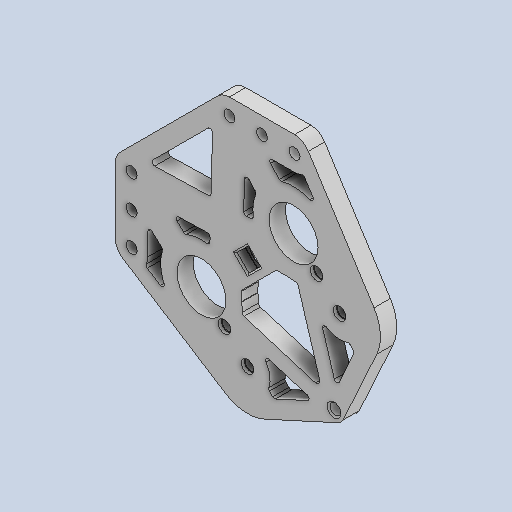
# Autodesk Inventor part: motorplate
Saved by Autodesk Inventor 2022 (Build 260153000, 153)
## iProperties
Created: 2022-03-17
Part Number: motorplate
Material: Generic
Document SubType Name: Modeling
Designer: zac-h
Density: 1 g/cm^3
Appearance: Default
Author: zac-h
## iProperties of the stored document motorplate_3DPrint.ipt
Created: 2022-03-19
Part Number: motorplate_3DPrint
Material: Generic
Document SubType Name: Modeling
Designer: zac-h
Density: 1 g/cm^3
Appearance: Default
Author: zac-h
Autodesk Inventor part; units mm, degrees
ref_plane "YZ Plane" through (0, 0, 0) normal (1, 0, 0) x (0, 1, 0)
ref_plane "XZ Plane" through (0, 0, 0) normal (0, 1, 0) x (-1, 0, 0)
ref_plane "XY Plane" through (0, 0, 0) normal (0, 0, 1) x (1, 0, 0)
sketch "Sketch1" plane through (0, 0, 0) normal (0, 0, 1) x (1, 0, 0)
  line L0 (-54.9162, 38.4967) -> (-54.9162, 12.4519) projected
  arc A0 (-54.9162, -18.4488) -> (-54.6412, -19.1376) centre (-53.9162, -18.4488) ccw projected
  line L1 (-54.6412, -19.1376) -> (-23.6992, -51.7087) projected
  arc A1 (-23.6992, -51.7087) -> (-14.0094, -54.6745) centre (-16.228, -44.6112) ccw projected
  line L2 (-14.0094, -54.6745) -> (-0.0667, -51.6007) projected
  arc A2 (-0.0667, -51.6007) -> (0.1266, -51.5369) centre (-0.282, -50.6241) ccw projected
  line L3 (0.1266, -51.5369) -> (17.6889, -43.6752) projected
  line L4 (43.6752, -17.6889) -> (51.5369, -0.1266) projected
  arc A3 (51.5369, -0.1266) -> (51.6007, 0.0667) centre (50.6241, 0.282) ccw projected
  line L5 (51.6007, 0.0667) -> (54.6745, 14.0094) projected
  arc A4 (54.6745, 14.0094) -> (51.7087, 23.6992) centre (44.6112, 16.228) ccw projected
  line L6 (51.7087, 23.6992) -> (19.1376, 54.6412) projected
  arc A5 (19.1376, 54.6412) -> (18.4488, 54.9162) centre (18.4488, 53.9162) ccw projected
  line L7 (0.0011, 54.9162) -> (-8.4105, 54.9162) projected
  circle A6 centre (14.5893, 21.3317) radius 9.525
  line L8 (-3.3712, 3.3712) -> (68.4985, -68.4985) construction
  circle A7 centre (30.3259, -30.3259) radius 3.8901
  line L9 (30.3259, -30.3259) -> (-3.3712, 3.3712) construction
  line L10 (14.5893, 21.3317) -> (32.5498, 3.3712) construction
  circle A8 centre (14.5893, 21.3317) radius 2.132
  circle A9 centre (23.5696, 12.3514) radius 2.132
  circle A10 centre (32.5498, 3.3712) radius 2.132
  line L11 (14.9688, 48.5312) -> (-10.4312, 48.5312) construction
  line L12 (14.9688, 42.1462) -> (-10.4312, 42.1462)
  line L13 (-10.4312, 54.9162) -> (14.9688, 54.9162)
  arc A11 (14.9688, 42.1462) -> (14.9688, 54.9162) centre (14.9688, 48.5312) ccw
  arc A12 (-10.4312, 54.9162) -> (-10.4312, 42.1462) centre (-10.4312, 48.5312) ccw
  line L14 (43.7752, 14.5965) -> (33.2607, 25.111)
  arc A13 (33.2607, 25.111) -> (-1.2806, 31.8696) centre (14.5893, 21.3317) ccw
  arc A14 (-1.2806, 31.8696) -> (-31.8696, 1.2806) centre (-3.3712, 3.3712) ccw
  arc A15 (-31.8696, 1.2806) -> (-25.111, -33.2607) centre (-21.3317, -14.5893) ccw
  line L15 (-25.111, -33.2607) -> (-14.5965, -43.7752)
  arc A16 (-14.5965, -43.7752) -> (8.8742, -22.4471) centre (-3.3712, -32.5498) ccw
  arc A17 (8.8742, -22.4471) -> (22.4471, -8.8742) centre (-3.3712, 3.3712) ccw
  arc A18 (22.4471, -8.8742) -> (43.7752, 14.5965) centre (32.5498, 3.3712) ccw
  line L16 (46.9883, -3.2279) -> (33.864, -31.943)
  line L17 (45.9291, 11.9158) -> (20.35, 51.9679)
  line L18 (-11.9158, -45.9291) -> (-51.9679, -20.35)
  circle A19 centre (-12.3514, -23.5696) radius 2.132
  circle A20 centre (-3.3712, -32.5498) radius 2.132
  arc A21 (-54.9162, -14.9688) -> (-42.1462, -14.9688) centre (-48.5312, -14.9688) ccw
  arc A22 (-42.1462, 10.4312) -> (-54.9162, 10.4312) centre (-48.5312, 10.4312) ccw
  line L19 (3.2279, -46.9883) -> (31.943, -33.864)
  line L20 (-53.0461, 14.9461) -> (-14.9461, 53.0461)
  circle A23 centre (-21.3317, -14.5893) radius 9.525
  arc A24 (17.6889, -43.6752) -> (30.0935, -35.8334) centre (-3.3712, 3.3712) ccw projected
  arc A25 (30.0935, -35.8334) -> (29.6251, -33.7616) centre (29.3145, -34.9207) ccw projected
  line L21 (29.6251, -33.7616) -> (27.4682, -33.1836) projected
  line L22 (27.4682, -33.1836) -> (26.4222, -29.2799) projected
  line L23 (26.4222, -29.2799) -> (29.2799, -26.4222) projected
  line L24 (29.2799, -26.4222) -> (33.1836, -27.4682) projected
  line L25 (33.1836, -27.4682) -> (33.7616, -29.6251) projected
  arc A26 (33.7616, -29.6251) -> (35.8334, -30.0935) centre (34.9207, -29.3145) ccw projected
  arc A27 (35.8334, -30.0935) -> (43.6752, -17.6889) centre (-3.3712, 3.3712) ccw projected
  arc A28 (7.8958, -33.0248) -> (33.0248, -7.8958) centre (-3.3712, 3.3712) ccw projected
  arc A29 (-10.1064, -39.285) -> (5.7833, -35.1808) centre (-3.3712, -32.5498) ccw projected
  line L26 (-10.1064, -39.285) -> (-16.8416, -32.5498) projected
  arc A30 (31.8591, 17.8778) -> (-17.8778, -31.8591) centre (-3.3712, 3.3712) ccw projected
  line L27 (32.5498, 16.8416) -> (39.285, 10.1064) projected
  arc A31 (35.1808, -5.7833) -> (39.285, 10.1064) centre (32.5498, 3.3712) ccw projected
  arc A32 (-38.4967, 54.9162) -> (-54.9162, 38.4967) centre (-38.4967, 38.4967) ccw projected
  arc A33 (-16.8416, -32.5498) -> (-17.8778, -31.8591) centre (-19.0866, -34.7949) ccw projected
  arc A34 (31.8591, 17.8778) -> (32.5498, 16.8416) centre (34.7949, 19.0866) ccw projected
  arc A35 (35.1808, -5.7833) -> (33.0248, -7.8958) centre (36.0578, -8.8347) ccw projected
  arc A36 (7.8958, -33.0248) -> (5.7833, -35.1808) centre (8.8347, -36.0578) ccw projected
  circle A37 centre (30.3259, -30.3259) radius 2.132
  line L28 (-8.4105, 54.9162) -> (-8.4105, 53.2312) projected
  line L29 (-8.4105, 53.2312) -> (-7.7176, 53.2312) projected
  line L30 (-7.7176, 53.2312) -> (-5.0041, 48.5312) projected
  line L31 (-5.0041, 48.5312) -> (-7.7176, 43.8312) projected
  line L32 (-7.7176, 43.8312) -> (-13.1447, 43.8312) projected
  line L33 (-13.1447, 43.8312) -> (-15.8583, 48.5312) projected
  line L34 (-15.8583, 48.5312) -> (-13.1447, 53.2312) projected
  line L35 (-13.1447, 53.2312) -> (-12.4519, 53.2312) projected
  line L36 (-12.4519, 53.2312) -> (-12.4519, 54.9162) projected
  line L37 (-12.4519, 54.9162) -> (-38.4967, 54.9162) projected
  line L38 (-54.9162, 12.4519) -> (-53.2312, 12.4519) projected
  line L39 (-53.2312, 12.4519) -> (-53.2312, 13.1447) projected
  line L40 (-53.2312, 13.1447) -> (-48.5312, 15.8583) projected
  line L41 (-48.5312, 15.8583) -> (-43.8312, 13.1447) projected
  line L42 (-43.8312, 13.1447) -> (-43.8312, 7.7176) projected
  line L43 (-43.8312, 7.7176) -> (-48.5312, 5.0041) projected
  line L44 (-48.5312, 5.0041) -> (-53.2312, 7.7176) projected
  line L45 (-53.2312, 7.7176) -> (-53.2312, 8.4105) projected
  line L46 (-53.2312, 8.4105) -> (-54.9162, 8.4105) projected
  line L47 (-54.9162, 8.4105) -> (-54.9162, -0.2481) projected
  line L48 (-54.9162, -0.2481) -> (-53.2312, -0.2481) projected
  line L49 (-53.2312, -0.2481) -> (-53.2312, 0.4447) projected
  line L50 (-53.2312, 0.4447) -> (-48.5312, 3.1583) projected
  line L51 (-48.5312, 3.1583) -> (-43.8312, 0.4447) projected
  line L52 (-43.8312, 0.4447) -> (-43.8312, -4.9824) projected
  line L53 (-43.8312, -4.9824) -> (-48.5312, -7.6959) projected
  line L54 (-48.5312, -7.6959) -> (-53.2312, -4.9824) projected
  line L55 (-53.2312, -4.9824) -> (-53.2312, -4.2895) projected
  line L56 (-53.2312, -4.2895) -> (-54.9162, -4.2895) projected
  line L57 (-54.9162, -4.2895) -> (-54.9162, -12.9481) projected
  line L58 (-54.9162, -12.9481) -> (-53.2312, -12.9481) projected
  line L59 (-53.2312, -12.9481) -> (-53.2312, -12.2553) projected
  line L60 (-53.2312, -12.2553) -> (-48.5312, -9.5417) projected
  line L61 (-48.5312, -9.5417) -> (-43.8312, -12.2553) projected
  line L62 (-43.8312, -12.2553) -> (-43.8312, -17.6824) projected
  line L63 (-43.8312, -17.6824) -> (-48.5312, -20.3959) projected
  line L64 (-48.5312, -20.3959) -> (-53.2312, -17.6824) projected
  line L65 (-53.2312, -17.6824) -> (-53.2312, -16.9895) projected
  line L66 (-53.2312, -16.9895) -> (-54.9162, -16.9895) projected
  line L67 (-54.9162, -16.9895) -> (-54.9162, -18.4488) projected
  line L68 (18.4488, 54.9162) -> (16.9895, 54.9162) projected
  line L69 (16.9895, 54.9162) -> (16.9895, 53.2312) projected
  line L70 (16.9895, 53.2312) -> (17.6824, 53.2312) projected
  line L71 (17.6824, 53.2312) -> (20.3959, 48.5312) projected
  line L72 (20.3959, 48.5312) -> (17.6824, 43.8312) projected
  line L73 (17.6824, 43.8312) -> (12.2553, 43.8312) projected
  line L74 (12.2553, 43.8312) -> (9.5417, 48.5312) projected
  line L75 (9.5417, 48.5312) -> (12.2553, 53.2312) projected
  line L76 (12.2553, 53.2312) -> (12.9481, 53.2312) projected
  line L77 (12.9481, 53.2312) -> (12.9481, 54.9162) projected
  line L78 (12.9481, 54.9162) -> (4.2895, 54.9162) projected
  line L79 (4.2895, 54.9162) -> (4.2895, 53.2312) projected
  line L80 (4.2895, 53.2312) -> (4.9824, 53.2312) projected
  line L81 (4.9824, 53.2312) -> (7.6959, 48.5312) projected
  line L82 (7.6959, 48.5312) -> (4.9824, 43.8312) projected
  line L83 (4.9824, 43.8312) -> (-0.4447, 43.8312) projected
  line L84 (-0.4447, 43.8312) -> (-3.1583, 48.5312) projected
  line L85 (-3.1583, 48.5312) -> (-0.4447, 53.2312) projected
  line L86 (-0.4447, 53.2312) -> (0.0011, 53.2312) projected
  line L87 (0.0011, 53.2312) -> (0.0011, 54.9162) projected
  circle A38 centre (14.9688, 48.5312) radius 2.132
  circle A39 centre (2.2688, 48.5312) radius 2.132
  circle A40 centre (-10.4312, 48.5312) radius 2.132
  circle A41 centre (-48.5312, 10.4312) radius 2.132
  circle A42 centre (-48.5312, -14.9688) radius 2.1673
  circle A43 centre (-48.5312, -2.2688) radius 2.1673
  line L88 (-54.9162, -16.9895) -> (-54.9162, -12.9481)
  line L89 (-54.9162, -4.2895) -> (-54.9162, 10.4312)
  line L90 (16.9895, 54.9162) -> (-12.4519, 54.9162)
  line L91 (-54.9162, 12.5632) -> (-54.9162, 10.4312)
  point P0 (0, 0)
  point P1 (-54.9162, 10.4312)
  point P2 (-3.3712, 3.3712)
  point P3 (-3.3712, 3.3712)
  point P4 (16.9895, 54.588)
  point P5 (-12.4519, 54.588)
  point P6 (30.454, -34.5445)
  point P7 (34.5445, -30.454)
  point P8 (-54.588, -16.9895)
  point P9 (-54.588, 12.4519)
  dimension "d9" = 19.05
  dimension "d16" = 4.264
  dimension "d19" = 12.7
  dimension "d57" = 4.264
  dimension "d61" = 4.264
  dimension "d62" = 4.264
  constraints: 36 end point, 25 point on circle, 24 centre point, 13 symmetric about line, 12 tangent, 7 coincident, 3 collinear, 2 vertical, 1 horizontal, 1 midpoint, 1 parallel, 1 point on line, 14 other
  measures "d9" diameter of A6
  measures "d16" diameter of A8
  measures "d19" distance of A8.centre A9.centre
  measures "d57" diameter of A37
  measures "d61" diameter of A38
  measures "d62" diameter of A41
extrude "Extrusion1" add sketch "Sketch1" along normal blind 6.35 contours L38 L39 L40 L41 L42 L43 L44 L45 L46 L89 A22 | A22 L20 A12 L12 A11 L17 A18 L14 A13 A30 A15 L15 A16 L18 A21 L66 L65 L64 L63 L62 L61 L60 L59 L58 L57 L56 L55 L54 L53 L52 L51 L50 L49 L48 L47 L46 L45 L44 L43 L42 L41 L40 L39 L38 | L36 L35 L34 L33 L32 L31 L30 L29 L28 L7 L87 L86 L85 L84 L83 L82 L81 L80 L79 L13 L77 L76 L75 L74 L73 L72 L71 L70 L69 A11 L12 A12 | A12 L13 L28 L29 L30 L31 L32 L33 L34 L35 L36 | L48 L49 L50 L51 L52 L53 L54 L55 L56 L89 | L13 L79 L80 L81 L82 L83 L84 L85 L86 L87 | L58 L59 L60 L61 L62 L63 L64 L65 L66 A21 L88 | L13 A11 L69 L70 L71 L72 L73 L74 L75 L76 L77 | A18 A28 A35 A31 L27 A34 A30 A13 L14 | L16 A26 A7 L25 L24 L23 L22 L21 A25 L19 A16 A28 A18 | A28 A16 A17 A18 | A18 A17 A16 A28 A36 A29 L26 A33 A30 A15 A14 A13 A34 L27 A31 A35 | L16 A7 A26 | A16 L15 A15 A30 A33 L26 A29 A36 A28 | A7 A25 L21 L22 L23 L24 L25 A26 | A26 L25 A7 | A13 A14 A15 A30 | L19 A25 A7 | A7 L24 L25 | A7 L21 A25 | L24 A7 | L21 L22 A7 | A7 L23 L24 | A7 L22 | L23 A7 | L22 L23 A7
sketch "Sketch2" plane through (0, 0, 6.35) normal (0, 0, 1) x (1, 0, 0)
  circle A0 centre (-48.5312, -14.9688) radius 2.132 projected
  arc A1 (20.35, 51.9679) -> (14.9688, 54.9162) centre (14.9688, 48.5312) ccw projected
  arc A2 (-54.9162, -14.9688) -> (-51.9679, -20.35) centre (-48.5312, -14.9688) ccw projected
  line L0 (-51.9679, -20.35) -> (-11.9158, -45.9291) projected
  arc A3 (-11.9158, -45.9291) -> (3.2279, -46.9883) centre (-3.3712, -32.5498) ccw projected
  line L1 (3.2279, -46.9883) -> (31.943, -33.864) projected
  arc A4 (31.943, -33.864) -> (33.864, -31.943) centre (30.3259, -30.3259) ccw projected
  line L2 (33.864, -31.943) -> (46.9883, -3.2279) projected
  arc A5 (46.9883, -3.2279) -> (45.9291, 11.9158) centre (32.5498, 3.3712) ccw projected
  line L3 (45.9291, 11.9158) -> (20.35, 51.9679) projected
  circle A6 centre (-21.3317, -14.5893) radius 9.525 projected
  circle A7 centre (-3.3712, -32.5498) radius 2.132 projected
  circle A8 centre (-12.3514, -23.5696) radius 2.132 projected
  circle A9 centre (32.5498, 3.3712) radius 2.132 projected
  circle A10 centre (23.5696, 12.3514) radius 2.132 projected
  circle A11 centre (14.5893, 21.3317) radius 9.525 projected
  circle A12 centre (32.5498, 3.3712) radius 2.4614
  circle A13 centre (23.5696, 12.3514) radius 2.4614
  circle A14 centre (-3.3712, -32.5498) radius 2.132 projected
  circle A15 centre (-3.3712, -32.5498) radius 2.4614
  circle A16 centre (-12.3514, -23.5696) radius 2.4614
  line L4 (14.9688, 54.9162) -> (-10.4312, 54.9162) projected
  arc A17 (-10.4312, 54.9162) -> (-14.9461, 53.0461) centre (-10.4312, 48.5312) ccw projected
  line L5 (-14.9461, 53.0461) -> (-53.0461, 14.9461) projected
  arc A18 (-53.0461, 14.9461) -> (-54.9162, 10.4312) centre (-48.5312, 10.4312) ccw projected
  line L6 (-54.9162, 10.4312) -> (-54.9162, -14.9688) projected
  dimension "d26" = 4.9228
  constraints: 4 centre point, 4 coincident, 3 equal radius
  measures "d26" diameter of A12
extrude "Extrusion2" cut sketch "Sketch2" against normal blind 1.27 contours A7 | A8 | A9 | A10 | A12 | A13 | A15 | A16
sketch "Sketch3" plane through (0, 0, 6.35) normal (0, 0, 1) x (1, 0, 0)
  circle A0 centre (32.5498, 3.3712) radius 2.4614 projected
  circle A1 centre (-12.3514, -23.5696) radius 2.4614 projected
  circle A2 centre (23.5696, 12.3514) radius 2.4614 projected
  circle A3 centre (-3.3712, -32.5498) radius 2.4614 projected
  arc A4 (20.35, 51.9679) -> (14.9688, 54.9162) centre (14.9688, 48.5312) ccw projected
  arc A5 (-54.9162, -14.9688) -> (-51.9679, -20.35) centre (-48.5312, -14.9688) ccw projected
  line L0 (-51.9679, -20.35) -> (-11.9158, -45.9291) projected
  arc A6 (-11.9158, -45.9291) -> (3.2279, -46.9883) centre (-3.3712, -32.5498) ccw projected
  line L1 (3.2279, -46.9883) -> (31.943, -33.864) projected
  arc A7 (31.943, -33.864) -> (33.864, -31.943) centre (30.3259, -30.3259) ccw projected
  line L2 (33.864, -31.943) -> (46.9883, -3.2279) projected
  arc A8 (46.9883, -3.2279) -> (45.9291, 11.9158) centre (32.5498, 3.3712) ccw projected
  line L3 (45.9291, 11.9158) -> (20.35, 51.9679) projected
  circle A9 centre (-21.3317, -14.5893) radius 9.525 projected
  circle A10 centre (14.5893, 21.3317) radius 9.525 projected
  line L4 (-48.5559, 10.4559) -> (-10.4559, 48.5559)
  arc A11 (-10.4312, 48.5662) -> (-10.4559, 48.5559) centre (-10.4312, 48.5312) ccw
  line L5 (-10.4312, 48.5662) -> (14.9688, 48.5662)
  arc A12 (14.9983, 48.55) -> (14.9688, 48.5662) centre (14.9688, 48.5312) ccw
  line L6 (14.9983, 48.55) -> (40.5774, 8.498)
  arc A13 (41.2129, -0.5883) -> (40.5774, 8.498) centre (32.5498, 3.3712) ccw
  line L7 (41.2129, -0.5883) -> (28.4697, -28.4697)
  line L8 (28.4697, -28.4697) -> (0.5883, -41.2129)
  arc A14 (-8.498, -40.5774) -> (0.5883, -41.2129) centre (-3.3712, -32.5498) ccw
  line L9 (-8.498, -40.5774) -> (-48.55, -14.9983)
  arc A15 (-48.5662, -14.9688) -> (-48.55, -14.9983) centre (-48.5312, -14.9688) ccw
  line L10 (-48.5662, -14.9688) -> (-48.5662, 10.4312)
  arc A16 (-48.5559, 10.4559) -> (-48.5662, 10.4312) centre (-48.5312, 10.4312) ccw
  line L11 (-48.5662, 10.4312) -> (-48.5662, -14.9688) construction
  line L12 (-54.9162, 10.4312) -> (-54.9162, -14.9688)
  line L13 (-42.2162, -14.9688) -> (-42.2162, 10.4312)
  arc A17 (-42.2162, 10.4312) -> (-54.9162, 10.4312) centre (-48.5662, 10.4312) ccw
  arc A18 (-54.9162, -14.9688) -> (-42.2162, -14.9688) centre (-48.5662, -14.9688) ccw
  circle A19 centre (-21.3317, -14.5893) radius 15.875
  circle A20 centre (-12.3514, -23.5696) radius 8.8114
  circle A21 centre (-3.3712, -32.5498) radius 8.8114
  circle A22 centre (30.3259, -30.3259) radius 8.482
  circle A23 centre (32.5498, 3.3712) radius 8.8114
  circle A24 centre (23.5696, 12.3514) radius 8.8114
  circle A25 centre (14.5893, 21.3317) radius 15.875
  circle A26 centre (-10.4312, 48.5312) radius 2.132 projected
  circle A27 centre (14.9688, 48.5312) radius 2.132 projected
  line L14 (-10.4312, 48.5312) -> (14.9688, 48.5312) construction
  line L15 (-10.4312, 42.1812) -> (14.9688, 42.1812)
  line L16 (14.9688, 54.8812) -> (-10.4312, 54.8812)
  arc A28 (-10.4312, 54.8812) -> (-10.4312, 42.1812) centre (-10.4312, 48.5312) ccw
  arc A29 (14.9688, 42.1812) -> (14.9688, 54.8812) centre (14.9688, 48.5312) ccw
  line L17 (-21.3317, -14.5893) -> (14.5893, 21.3317) construction
  line L18 (-16.8416, -19.0795) -> (19.0795, 16.8416)
  line L19 (10.0992, 25.8218) -> (-25.8218, -10.0992)
  arc A30 (-25.8218, -10.0992) -> (-16.8416, -19.0795) centre (-21.3317, -14.5893) ccw
  arc A31 (19.0795, 16.8416) -> (10.0992, 25.8218) centre (14.5893, 21.3317) ccw
  line L20 (14.5893, 21.3317) -> (66.3854, -30.4643) construction
  line L21 (12.3443, 19.0866) -> (64.1403, -32.7094)
  line L22 (68.6304, -28.2193) -> (16.8344, 23.5768)
  arc A32 (16.8344, 23.5768) -> (12.3443, 19.0866) centre (14.5893, 21.3317) ccw
  arc A33 (64.1403, -32.7094) -> (68.6304, -28.2193) centre (66.3854, -30.4643) ccw
  line L23 (14.5893, 21.3317) -> (87.84, 21.3317) construction
  line L24 (-21.3317, -14.5893) -> (30.4643, -66.3854) construction
  line L25 (-23.5768, -16.8344) -> (28.2193, -68.6304)
  line L26 (32.7094, -64.1403) -> (-19.0866, -12.3443)
  arc A34 (-19.0866, -12.3443) -> (-23.5768, -16.8344) centre (-21.3317, -14.5893) ccw
  arc A35 (28.2193, -68.6304) -> (32.7094, -64.1403) centre (30.4643, -66.3854) ccw
  line L27 (-21.3317, -14.5893) -> (51.9189, -14.5893) construction
  line L28 (14.5893, 21.3317) -> (-10.4312, 48.5312) construction
  line L29 (19.2627, 25.6307) -> (-5.7578, 52.8302)
  line L30 (-15.1046, 44.2322) -> (9.9159, 17.0327)
  arc A36 (9.9159, 17.0327) -> (19.2627, 25.6307) centre (14.5893, 21.3317) ccw
  arc A37 (-5.7578, 52.8302) -> (-15.1046, 44.2322) centre (-10.4312, 48.5312) ccw
  line L31 (-21.3317, -14.5893) -> (-48.5662, 10.4312) construction
  line L32 (-17.0357, -9.9132) -> (-44.2701, 15.1074)
  line L33 (-52.8622, 5.755) -> (-25.6277, -19.2655)
  arc A38 (-25.6277, -19.2655) -> (-17.0357, -9.9132) centre (-21.3317, -14.5893) ccw
  arc A39 (-44.2701, 15.1074) -> (-52.8622, 5.755) centre (-48.5662, 10.4312) ccw
  circle A40 centre (30.3259, -30.3259) radius 2.132 projected
  line L34 (30.3259, -30.3259) -> (14.5893, 21.3317) construction
  line L35 (33.3631, -29.4007) -> (17.6265, 22.2569)
  line L36 (11.5521, 20.4065) -> (27.2887, -31.2511)
  arc A41 (27.2887, -31.2511) -> (33.3631, -29.4007) centre (30.3259, -30.3259) ccw
  arc A42 (17.6265, 22.2569) -> (11.5521, 20.4065) centre (14.5893, 21.3317) ccw
  line L37 (-21.3317, -14.5893) -> (30.3259, -30.3259) construction
  line L38 (-22.2569, -17.6265) -> (29.4007, -33.3631)
  line L39 (31.2511, -27.2887) -> (-20.4065, -11.5521)
  arc A43 (-20.4065, -11.5521) -> (-22.2569, -17.6265) centre (-21.3317, -14.5893) ccw
  arc A44 (29.4007, -33.3631) -> (31.2511, -27.2887) centre (30.3259, -30.3259) ccw
  circle A45 centre (-48.5312, 10.4312) radius 2.132 projected
  circle A46 centre (23.5696, 12.3514) radius 2.132 projected
  line L40 (-48.5312, 10.4312) -> (23.5696, 12.3514) construction
  line L41 (-48.3621, 4.0834) -> (23.7386, 6.0037)
  line L42 (23.4005, 18.6992) -> (-48.7002, 16.7789)
  arc A47 (-48.7002, 16.7789) -> (-48.3621, 4.0834) centre (-48.5312, 10.4312) ccw
  arc A48 (23.7386, 6.0037) -> (23.4005, 18.6992) centre (23.5696, 12.3514) ccw
  circle A49 centre (-12.3514, -23.5696) radius 2.132 projected
  line L43 (-10.4312, 48.5312) -> (-12.3514, -23.5696) construction
  line L44 (-16.7789, 48.7002) -> (-18.6992, -23.4005)
  line L45 (-6.0037, -23.7386) -> (-4.0834, 48.3621)
  arc A50 (-4.0834, 48.3621) -> (-16.7789, 48.7002) centre (-10.4312, 48.5312) ccw
  arc A51 (-18.6992, -23.4005) -> (-6.0037, -23.7386) centre (-12.3514, -23.5696) ccw
  line L46 (14.9688, 54.9162) -> (-10.4312, 54.9162) projected
  arc A52 (-10.4312, 54.9162) -> (-14.9461, 53.0461) centre (-10.4312, 48.5312) ccw projected
  line L47 (-14.9461, 53.0461) -> (-53.0461, 14.9461) projected
  arc A53 (-53.0461, 14.9461) -> (-54.9162, 10.4312) centre (-48.5312, 10.4312) ccw projected
  line L48 (-54.9162, 10.4312) -> (-54.9162, -14.9688) projected
  point P0 (0, 0)
  point P1 (-48.5662, -2.2688)
  point P2 (2.2688, 48.5312)
  point P3 (-3.3712, 3.3712)
  point P4 (40.4873, -4.5663)
  point P5 (4.5663, -40.4873)
  point P6 (2.0791, 34.9314)
  point P7 (-34.9489, -2.0791)
  point P8 (22.4576, -4.4971)
  point P9 (4.4971, -22.4576)
  point P10 (-12.4808, 11.3913)
  point P11 (-11.3913, 12.4808)
  point P12 (-18.0508, 0.9429)
  point P13 (-17.9456, 4.8935)
  point P14 (-32.7241, 4.4999)
  point P15 (-27.7501, -0.0697)
  point P16 (-36.3422, -9.4221)
  point P17 (-42.2162, -4.0256)
  point P18 (-43.2232, -18.4003)
  point P19 (-33.7957, -24.4211)
  point P20 (4.0382, 42.1812)
  point P21 (9.4124, 36.3389)
  point P22 (24.4211, 33.7957)
  point P23 (18.4161, 43.1984)
  point P24 (-4.5004, 32.7045)
  point P25 (-4.8935, 17.9456)
  point P26 (-0.9429, 18.0508)
  point P27 (0.0656, 27.7408)
  point P28 (-17.607, 17.607)
  point P29 (-16.9559, 42.056)
  point P30 (-42.056, 16.9559)
  point P31 (24.4007, 0.0198)
  point P32 (31.0711, -21.8767)
  point P33 (31.463, -21.9205)
  point P34 (38.329, -6.8981)
  point P35 (36.1168, -4.6859)
  point P36 (21.8767, -31.0711)
  point P37 (-0.0198, -24.4007)
  point P38 (4.6859, -36.1168)
  point P39 (6.8981, -38.329)
  point P40 (21.9205, -31.463)
  point P41 (-5.5797, -7.8176)
  point P42 (-5.6881, -11.8887)
  point P43 (-5.5273, -16.0848)
  point P44 (23.7272, -24.9967)
  point P45 (24.9967, -23.7272)
  point P46 (16.0848, 5.5273)
  point P47 (11.8887, 5.6881)
  point P48 (7.8176, 5.5797)
  dimension "d28" = 12.7
  dimension "d29" = 6.35
  dimension "d30" = 6.35
  dimension "d31" = 6.35
  dimension "d33" = 12.7
  dimension "d34" = 12.7
  dimension "d35" = 45
  dimension "d36" = 6.35
  dimension "d37" = 45
  dimension "d38" = 6.35
  dimension "d39" = 12.7
  dimension "d40" = 12.7
  dimension "d41" = 6.35
  dimension "d42" = 6.35
  dimension "d43" = 12.7
  dimension "d44" = 12.7
  constraints: 106 end point, 56 point on circle, 44 tangent, 35 centre point, 14 equal length, 11 midpoint, 6 equal radius, 3 horizontal, 7 other
  measures "d28" diameter of A18
  measures "d29" radial gap between concentric circles of A9 A19
  measures "d30" radial gap between concentric circles of A1 A20
  measures "d31" radial gap between concentric circles of A3 A21
  measures "d33" diameter of A29
  measures "d34" diameter of A31
  measures "d35" angle of L20 L23
  measures "d36" diameter of A33
  measures "d37" angle of L24 L27
  measures "d38" diameter of A35
  measures "d39" diameter of A37
  measures "d40" diameter of A39
  measures "d41" diameter of A42
  measures "d42" diameter of A44
  measures "d43" diameter of A48
  measures "d44" diameter of A51
extrude "Extrusion3" cut sketch "Sketch3" against normal through all contours L7 A22 L35 A23 L21 | A18 L13 L33 A19 L9 | L4 L44 L42 | L8 L26 A21 L38 A22 | A22 L39 A19 L45 L18 L41 A25 L36 | A25 L29 L15 A29 L6 | L41 L44 A19 L32 | L45 L30 A25 L42
fillet "Fillet1" radius 1 37 edges at (24.4007, 0.0198, 3.175) (31.0711, -21.8767, 3.175) (31.463, -21.9205, 3.175) (38.329, -6.8981, 3.175) (36.1168, -4.6859, 3.175) (-36.3422, -9.4221, 3.175) (-42.2162, -4.0256, 3.175) (-43.2232, -18.4003, 3.175) (-33.7957, -24.4211, 3.175) (4.0382, 42.1812, 3.175) (9.4124, 36.3389, 3.175) (24.4211, 33.7957, 3.175) (18.4161, 43.1984, 3.175) (21.8767, -31.0711, 3.175) (-0.0198, -24.4007, 3.175) (4.6859, -36.1168, 3.175) (6.8981, -38.329, 3.175) (21.9205, -31.463, 3.175) (-16.9559, 42.056, 3.175) (-42.056, 16.9559, 3.175) (-17.607, 17.607, 3.175) (-18.0508, 0.9429, 3.175) (-17.9456, 4.8935, 3.175) (-32.7241, 4.4999, 3.175) (-27.7501, -0.0697, 3.175) (-4.5004, 32.7045, 3.175) (-4.8935, 17.9456, 3.175) (-0.9429, 18.0508, 3.175) (0.0656, 27.7408, 3.175) (11.8887, 5.6881, 3.175) (7.8176, 5.5797, 3.175) (-5.5797, -7.8176, 3.175) (-5.6881, -11.8887, 3.175) (-5.5273, -16.0848, 3.175) (23.7272, -24.9967, 3.175) (24.9967, -23.7272, 3.175) (16.0848, 5.5273, 3.175)
sketch "Sketch4" plane through (0, 0, 0) normal (0, 0, -1) x (-1, 0, 0)
  circle A0 centre (3.3712, 3.3712) radius 38.025 projected
  line L0 (8.0593, 3.3712) -> (3.3712, 8.0593)
  line L1 (3.3712, 8.0593) -> (-1.3169, 3.3712)
  line L2 (-1.3169, 3.3712) -> (3.3712, -1.3169)
  line L3 (3.3712, -1.3169) -> (8.0593, 3.3712)
  line L4 (8.0593, 3.3712) -> (-1.3169, 3.3712) construction
  line L5 (3.3712, 8.0593) -> (3.3712, -1.3169) construction
  point P0 (0, 0)
  dimension "d48" = 6.63
  constraints: 12 end point, 2 midpoint, 2 parallel, 2 perpendicular, 1 vertical
  measures "d48" distance of L0.end L1.end
extrude "Extrusion4" cut sketch "Sketch4" against normal blind 25.4 contours L3 L2 L1 L0
sketch "Sketch5" plane through (0, 0, 0) normal (0, 0, -1) x (-1, 0, 0)
  line L0 (3.3712, -1.3169) -> (8.0593, 3.3712) projected
  line L1 (-1.3169, 3.3712) -> (3.3712, -1.3169) projected
  line L2 (3.3712, 8.0593) -> (-1.3169, 3.3712) projected
  line L3 (8.0593, 3.3712) -> (3.3712, 8.0593) projected
  line L4 (8.0593, 3.3712) -> (3.3712, -1.3169) projected
  line L5 (3.3712, 8.0593) -> (8.0593, 3.3712) projected
  line L6 (3.3712, -1.3169) -> (3.3712, 8.0593) construction
  line L7 (3.3712, -1.3169) -> (-1.3169, 3.3712) projected
  line L8 (-1.3169, 3.3712) -> (8.0593, 3.3712) construction
  circle A0 centre (3.3712, 3.3712) radius 5.025
  point P0 (0, 0)
  dimension "d51" = 10.05
  constraints: 4 end point, 1 centre point, 1 horizontal, 1 midpoint, 1 vertical
  measures "d51" diameter of A0
extrude "Extrusion5" cut sketch "Sketch5" against normal blind 2 contours L1 L2 L3 L0 | A0
chamfer "Chamfer1" distance 0.6 angle 45 9 edges at (1.6538, 3.3712, 0) (-1.0271, 1.0271, 2) (-5.7152, 1.0271, 2) (-5.7152, 5.7152, 2) (-1.0271, 5.7152, 2) (-1.0271, 5.7152, 6.35) (-1.0271, 1.0271, 6.35) (-5.7152, 1.0271, 6.35) (-5.7152, 5.7152, 6.35)
chamfer "Chamfer2" distance 0.6 angle 45 1 edges at (28.1939, -30.3259, 6.35)
body "Solid1"
